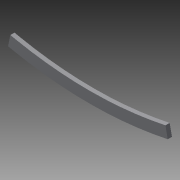
# Autodesk Inventor part: nd-k
Saved by Autodesk Inventor 2015 (Build 190159000, 159)
## iProperties
Created: 2014-07-02
Part Number: nd-k
Material: Generic
Document SubType Name: Modeling
Designer: peter
Density: 1 g/cm^3
Appearance: Default
Author: peter
Autodesk Inventor part; units mm, degrees
ref_plane "YZ Plane" through (0, 0, 0) normal (1, 0, 0) x (0, 1, 0)
ref_plane "XZ Plane" through (0, 0, 0) normal (0, 1, 0) x (-1, 0, 0)
ref_plane "XY Plane" through (0, 0, 0) normal (0, 0, 1) x (1, 0, 0)
sketch "Sketch1" plane through (0, 0, 0) normal (0, 0, 1) x (1, 0, 0)
  line L0 (10.3699, 89.9779) -> (35.2697, 84.7858)
  arc A0 (35.2697, 84.7858) -> (718.8116, 87.08) centre (371.5322, 1727.1148) ccw
  line L1 (718.8116, 87.08) -> (729.3349, 37.3834)
  arc A1 (25.08, 35.0183) -> (729.3349, 37.3834) centre (371.5288, 1727.0806) ccw
  line L2 (25.08, 35.0183) -> (24.99, 35.0367)
  line L3 (24.99, 35.0367) -> (0.0002, 40.2475)
  line L4 (0.0002, 40.2475) -> (10.3699, 89.9779)
  point P0 (0, 0)
  constraints: 10 end point, 4 point on circle, 2 centre point
extrude "Extrusion1" add sketch "Sketch1" along normal blind 19.05
body "Solid1"
